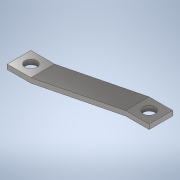
# Autodesk Inventor part: Docisk_sprężynka
Saved by Autodesk Inventor 2022 (Build 260153000, 153)
## iProperties
Created: 2021-05-23
Part Number: Docisk_sprężynka
Material: Stal, węglowa
Document SubType Name: Modeling
Designer: Matik
Density: 7.85 g/cm^3
Appearance: Częściowo polerowany
Author: Matik
Autodesk Inventor part; units mm, degrees
ref_plane "YZ Plane" through (0, 0, 0) normal (1, 0, 0) x (0, 1, 0)
ref_plane "XZ Plane" through (0, 0, 0) normal (0, 1, 0) x (-1, 0, 0)
ref_plane "XY Plane" through (0, 0, 0) normal (0, 0, 1) x (1, 0, 0)
sketch "Szkic1" plane through (0, 0, 0) normal (0, 0, 1) x (1, 0, 0)
  line L0 (-35.4869, -5) -> (-25.4869, -5)
  line L1 (-25.4869, -3) -> (-35.4869, -3)
  line L2 (-35.4869, -5) -> (-35.4869, -3)
  line L3 (24.5131, 5) -> (14.5131, 5)
  line L4 (24.5131, 3) -> (24.5131, 3)
  line L5 (24.5131, 3) -> (24.5131, 5)
  line L6 (24.5131, 3) -> (14.5131, 3)
  line L7 (14.5131, 3) -> (-25.4869, -5)
  line L8 (-25.4869, -3) -> (14.5131, 5)
  point P0 (24.5131, 5)
  dimension "d9" = 10
  dimension "d10" = 2
  dimension "d11" = 10
  dimension "d14" = 60
  dimension "d15" = 10
  constraints: 18 end point, 3 horizontal, 2 vertical, 1 parallel, 1 point on line
  measures "d9" distance of L1.start L1.end
  measures "d10" distance of L4.end L3.start
  measures "d11" distance of L3.start L3.end
  measures "d14" horizontal distance of L4.end L0.start
  measures "d15" distance of L4.end L6.end
extrude "Wyciągnięcie proste1" add sketch "Szkic1" along normal blind 10
sketch "Szkic2" plane through (-35.4869, -3, 0) normal (0, 1, 0) x (1, 0, 0)
  line L0 (10, 0) -> (10, -10) projected
  line L1 (10, -5) -> (0, -5)
  line L2 (0, 0) -> (0, -10) projected
  circle A0 centre (5, -5) radius 2.5
  point P0 (35.4869, 0)
  dimension "d16" = 5
  constraints: 3 midpoint, 2 end point, 1 centre point
  measures "d16" diameter of A0
extrude "Wyciągnięcie proste2" cut sketch "Szkic2" against normal blind 10
sketch "Szkic3" plane through (14.5131, 5, 0) normal (0, 1, 0) x (1, 0, 0)
  line L0 (10, 0) -> (10, -10) projected
  line L1 (10, -5) -> (0, -5)
  line L2 (0, 0) -> (0, -10) projected
  circle A0 centre (5, -5) radius 2.5
  point P0 (-14.5131, 0)
  dimension "d19" = 5
  constraints: 3 midpoint, 2 end point, 1 centre point
  measures "d19" diameter of A0
extrude "Wyciągnięcie proste3" cut sketch "Szkic3" against normal blind 10
